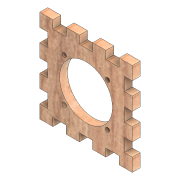
# Autodesk Inventor part: joystick behuizing boevnzijde
Saved by Autodesk Inventor 2020.3 (Build 243373000, 373)
## iProperties
Created: 2020-12-09
Part Number: joystick behuizing boevnzijde
Material: Wood (Birch)
Document SubType Name: Sheet Metal
Designer: Svend
Density: 0.55 g/cm^3
Sheet Metal Rule: Default
Appearance: Birch - Natural Polished
Author: Svend
Autodesk Inventor part; units mm, degrees
ref_plane "YZ Plane" through (0, 0, 0) normal (1, 0, 0) x (0, 1, 0)
ref_plane "XZ Plane" through (0, 0, 0) normal (0, 1, 0) x (-1, 0, 0)
ref_plane "XY Plane" through (0, 0, 0) normal (0, 0, 1) x (1, 0, 0)
sketch "Sketch1" plane through (0, 0, 0) normal (0, 0, 1) x (1, 0, 0)
  circle A0 centre (0, 0) radius 20
  line L0 (-35, 35) -> (35, 35)
  line L1 (35, 35) -> (35, -35)
  line L2 (35, -35) -> (-35, -35)
  line L3 (-35, -35) -> (-35, 35)
  line L4 (-35, 35) -> (35, -35) construction
  line L5 (35, 35) -> (-35, -35) construction
  circle A1 centre (-16.35, 16.35) radius 1.6
  circle A2 centre (16.35, 16.35) radius 1.6
  circle A3 centre (-16.35, -16.35) radius 1.6
  circle A4 centre (16.35, -16.35) radius 1.6
  line L6 (35, 5) -> (29, 5)
  line L7 (29, 5) -> (29, -5)
  line L8 (29, -5) -> (35, -5)
  line L9 (35, -5) -> (35, 5)
  line L10 (35, -15) -> (29, -15)
  line L11 (29, -25) -> (35, -25)
  line L12 (29, -15) -> (29, -25)
  line L13 (35, -25) -> (35, -15)
  line L14 (35, 25) -> (29, 25)
  line L15 (29, 15) -> (35, 15)
  line L16 (29, 25) -> (29, 15)
  line L17 (35, 15) -> (35, 25)
  line L18 (35, 5) -> (29, 5)
  line L19 (29, -5) -> (35, -5)
  line L20 (29, 5) -> (29, -5)
  line L21 (35, -5) -> (35, 5)
  line L22 (0, 35) -> (0, -35) construction
  line L23 (-35, 0) -> (35, 0) construction
  line L24 (5, 29) -> (5, 35)
  line L25 (5, 29) -> (5, 35)
  line L26 (-5, 29) -> (5, 29)
  line L27 (5, 35) -> (-5, 35)
  line L28 (15, 29) -> (25, 29)
  line L29 (25, 35) -> (15, 35)
  line L30 (-5, 35) -> (-5, 29)
  line L31 (-5, 35) -> (-5, 29)
  line L32 (25, 29) -> (25, 35)
  line L33 (-5, 29) -> (5, 29)
  line L34 (15, 35) -> (15, 29)
  line L35 (5, 35) -> (-5, 35)
  line L36 (-15, 29) -> (-15, 35)
  line L37 (-25, 35) -> (-25, 29)
  line L38 (-15, 35) -> (-25, 35)
  line L39 (-25, 29) -> (-15, 29)
  line L40 (-29, 5) -> (-35, 5)
  line L41 (-29, 5) -> (-35, 5)
  line L42 (-29, -5) -> (-29, 5)
  line L43 (-35, 5) -> (-35, -5)
  line L44 (-29, 15) -> (-29, 25)
  line L45 (-35, 25) -> (-35, 15)
  line L46 (-35, -5) -> (-29, -5)
  line L47 (-35, -5) -> (-29, -5)
  line L48 (-29, 25) -> (-35, 25)
  line L49 (-29, -5) -> (-29, 5)
  line L50 (-35, 15) -> (-29, 15)
  line L51 (-35, 5) -> (-35, -5)
  line L52 (-29, -15) -> (-35, -15)
  line L53 (-35, -25) -> (-29, -25)
  line L54 (-35, -15) -> (-35, -25)
  line L55 (-29, -25) -> (-29, -15)
  line L56 (-5, -29) -> (-5, -35)
  line L57 (-5, -29) -> (-5, -35)
  line L58 (5, -29) -> (-5, -29)
  line L59 (-5, -35) -> (5, -35)
  line L60 (-15, -29) -> (-25, -29)
  line L61 (-25, -35) -> (-15, -35)
  line L62 (5, -35) -> (5, -29)
  line L63 (5, -35) -> (5, -29)
  line L64 (-25, -29) -> (-25, -35)
  line L65 (5, -29) -> (-5, -29)
  line L66 (-15, -35) -> (-15, -29)
  line L67 (-5, -35) -> (5, -35)
  line L68 (15, -29) -> (15, -35)
  line L69 (25, -35) -> (25, -29)
  line L70 (15, -35) -> (25, -35)
  line L71 (25, -29) -> (15, -29)
  point P0 (29, 0)
  point P1 (29, -20)
  point P2 (35, -20)
  point P3 (29, 20)
  point P4 (35, 20)
  point P5 (29, 0)
  point P6 (0, 29)
  point P7 (20, 35)
  point P8 (20, 29)
  point P9 (0, 29)
  point P10 (0, 35)
  point P11 (0, 35)
  point P12 (-20, 29)
  point P13 (-20, 35)
  point P14 (-29, 0)
  point P15 (-35, 20)
  point P16 (-29, 20)
  point P17 (-29, 0)
  point P18 (-35, 0)
  point P19 (-35, 0)
  point P20 (-29, -20)
  point P21 (-35, -20)
  point P22 (0, -29)
  point P23 (-20, -35)
  point P24 (-20, -29)
  point P25 (0, -29)
  point P26 (0, -35)
  point P27 (0, -35)
  point P28 (20, -29)
  point P29 (20, -35)
  dimension "d0" = 40
  dimension "d1" = 70
  dimension "d2" = 70
  dimension "d3" = 32.7
  dimension "d4" = 3.2
  dimension "d5" = 6
  dimension "d6" = 10
  dimension "d9" = 20
  dimension "d12" = 20
  dimension "d17" = 360
  constraints: 144 end point, 7 midpoint, 5 centre point, 5 point on line, 4 parallel, 3 equal radius, 2 horizontal, 2 horizontal alignment, 2 perpendicular, 2 vertical, 2 vertical alignment, 1 coincident, 191 other
  measures "d0" diameter of A0
  measures "d1" distance of L1.end L2.end
  measures "d2" distance of L0.end L1.end
  measures "d3" distance of A1.centre A2.centre
  measures "d4" diameter of A2
  measures "d5" distance of L8.end L7.end
  measures "d6" distance of L7.end L6.end
  measures "d9" distance of L6.start L10.start
  measures "d12" distance of L6.start L14.start
extrude "Extrusion1" add sketch "Sketch1" along normal blind 6 contours L0 L37 L39 L36 L30 L26 L24 L34 L28 L32 L1 L14 L16 L15 L6 L7 L8 L10 L12 L11 L2 L69 L71 L68 L62 L58 L56 L66 L60 L64 L3 L53 L55 L52 L46 L42 L40 L50 L44 L48
equation "\"d9\" = 2 * d6"
equation "\"d12\" = 2 * d6"
equation "\"BendRadius\" = Thickness"
equation "\"BendReliefWidth\" = Thickness"
equation "\"BendReliefDepth\" = 0.5 * Thickness"
equation "\"CornerReliefSize\" = 4 * Thickness"
equation "\"MinimumRemnant\" = 2 * Thickness"
equation "\"TransitionRadius\" = BendRadius"
equation "\"JacobiRadiusSize\" = Thickness"
equation "\"GapSize\" = Thickness"
equation "\"Thickness\" = 0.5"
body "Solid1"
